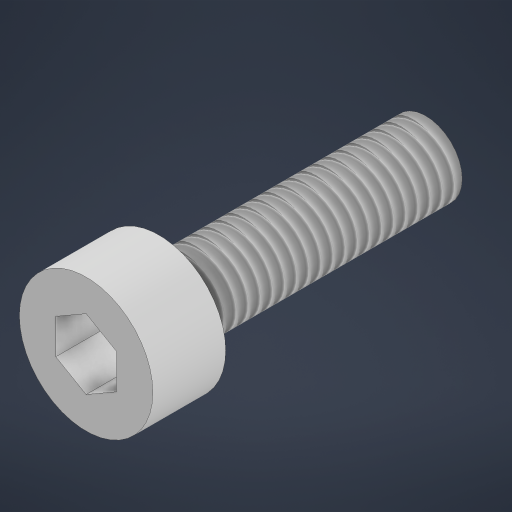
# Autodesk Inventor part: shaft
Saved by Autodesk Inventor 2023.5 (Build 275446000, 446)
## iProperties
Created: 2023-12-14
Part Number: shaft
Material: 一般
Document SubType Name: Modeling
Designer: IshiiLabHonda
Density: 1 g/cm^3
Appearance: 既定
Author: IshiiLabHonda
Autodesk Inventor part; units mm, degrees
ref_plane "YZ Plane" through (0, 0, 0) normal (1, 0, 0) x (0, 1, 0)
ref_plane "XZ Plane" through (0, 0, 0) normal (0, 1, 0) x (-1, 0, 0)
ref_plane "XY Plane" through (0, 0, 0) normal (0, 0, 1) x (1, 0, 0)
sketch "スケッチ1" plane through (0, 0, 0) normal (0, 0, 1) x (1, 0, 0)
  circle A0 centre (0, 0) radius 2.75
  circle A1 centre (0, 0) radius 1.25 construction
  line L0 (-1.25, 0.7217) -> (0, 1.4434)
  line L1 (0, 1.4434) -> (1.25, 0.7217)
  line L2 (1.25, 0.7217) -> (1.25, -0.7217)
  line L3 (1.25, -0.7217) -> (0, -1.4434)
  line L4 (0, -1.4434) -> (-1.25, -0.7217)
  line L5 (-1.25, -0.7217) -> (-1.25, 0.7217)
  point P0 (-1.25, 0)
  dimension "d1" = 2.5
  dimension "d0" = 5.5
  constraints: 12 end point, 3 coincident, 1 centre point, 1 horizontal alignment, 1 midpoint, 15 other
  measures "d0" diameter of A0
extrude "押し出し1" add sketch "スケッチ1" along normal blind 3
sketch "スケッチ2" plane through (0, 0, 0) normal (0, 0, 1) x (1, 0, 0)
  circle A0 centre (0, 0) radius 1.5
  dimension "d4" = 3
  constraints: 1 centre point, 1 coincident
  measures "d4" diameter of A0
extrude "押し出し2" add sketch "スケッチ2" against normal blind 11
thread "ねじ1" size "M3x0.5" class "6g" standard "ANSI Metric M Profile" length 11
